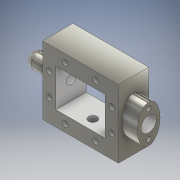
# Autodesk Inventor part: reverse gear steam chest
Saved by Autodesk Inventor 2017 (Build 210142000, 142)
## iProperties
Created: 2018-11-06
Part Number: reverse gear steam chest
Material: Generic
Document SubType Name: Modeling
Designer: User
Density: 1 g/cm^3
Appearance: Default
Author: User
Autodesk Inventor part; units mm, degrees
ref_plane "YZ Plane" through (0, 0, 0) normal (1, 0, 0) x (0, 1, 0)
ref_plane "XZ Plane" through (0, 0, 0) normal (0, 1, 0) x (-1, 0, 0)
ref_plane "XY Plane" through (0, 0, 0) normal (0, 0, 1) x (1, 0, 0)
sketch "Sketch1" plane through (0, 0, 0) normal (0, 1, 0) x (-1, 0, 0)
  line L0 (0, 0) -> (-40, 0)
  line L1 (-40, 0) -> (-40, -36)
  line L2 (-40, -36) -> (0, -36)
  line L3 (0, -36) -> (0, 0)
  line L4 (-7, -28) -> (-33, -28)
  line L5 (-33, -28) -> (-33, -8)
  line L6 (-33, -8) -> (-7, -8)
  line L7 (-7, -8) -> (-7, -28)
  dimension "d0" = 40
  dimension "d1" = 36
  dimension "d2" = 26
  constraints: 16 end point, 3 perpendicular, 2 parallel, 1 horizontal
  measures "d0" distance of L2.end L1.end
  measures "d1" distance of L1.end L0.end
  measures "d2" distance of L4.start L4.end
extrude "Extrusion1" add sketch "Sketch1" along normal blind 16
sketch "Sketch2" plane through (40, 0, 0) normal (1, 0, 0) x (0, 0, -1)
  line L0 (0, 0) -> (0, 16)
  line L1 (0, 8) -> (8, 8)
  line L2 (28, 0) -> (28, 16)
  line L3 (18, 14) -> (18, 2)
  ellipse E0 centre (18, 8) end of major axis (28, 8) minor radius 6
  line L4 (6.75, 0) -> (6.75, 16)
  line L5 (6.75, 8) -> (9.75, 8)
  circle A0 centre (11, 8) radius 1.25
  circle A1 centre (25, 8) radius 1.25
  circle A2 centre (18, 8) radius 2.5
  line L6 (12.25, 8) -> (15.5, 8)
  line L7 (20.5, 8) -> (23.75, 8)
  line L8 (20.5, 8) -> (23.75, 8)
  line L9 (26.25, 8) -> (28, 8)
  line L10 (8, 8) -> (9.75, 8)
  line L11 (12.25, 8) -> (15.5, 8)
  circle A3 centre (18, 8) radius 4
  line L12 (18, 8) -> (18, 10.5)
  line L13 (18, 12) -> (18, 14)
  dimension "d18" = 8
  dimension "d47" = 10
  dimension "d48" = 6
  dimension "d5" = 8
  dimension "d6" = 20
  dimension "d7" = 6
  dimension "d8" = 12
  dimension "d9" = 3
  dimension "d10" = 14
  dimension "d11" = 2.5
  dimension "d12" = 2.5
  dimension "d13" = 5
  dimension "d49" = 21.25
  dimension "d50" = 28
  dimension "d51" = 0
  dimension "d52" = 0
  dimension "d53" = 0
  dimension "d54" = 28
  dimension "d55" = 8
  dimension "d56" = 8
  dimension "d57" = 1.75
  dimension "d58" = 15.75
  dimension "d59" = 8
  dimension "d60" = 8
  dimension "d61" = 28
  dimension "d62" = 8
  constraints: 28 end point, 7 horizontal, 7 point on circle, 4 midpoint, 3 centre point, 3 parallel, 3 vertical, 2 coincident, 1 vertical alignment, 7 other
  measures "d5" distance of L1.start L1.end
  measures "d6" distance of L1.end L9.end
  measures "d7" distance of L12.start L3.start
  measures "d8" distance of L3.start L3.end
  measures "d9" distance of L5.start L5.end
  measures "d10" distance of L5.end L7.end
  measures "d11" diameter of A0
  measures "d12" diameter of A1
  measures "d13" diameter of A2
  measures "d49" distance between parallel lines of L4 L2
  measures "d50" distance between parallel lines of L0 L2
  measures "d51" distance between parallel lines of L9 L8
  measures "d52" distance between parallel lines of L9 L11
  measures "d53" distance between parallel lines of L1 L9
  measures "d54" distance from line of point (0, 0) L2
  measures "d55" distance from line of point (0, 0) L9
  measures "d56" distance from line of L2.end L9
  measures "d57" distance from line of L9.start L2
  measures "d58" distance from line of L6.start L2
  measures "d59" distance from line of L4.end L9
  measures "d60" distance from line of L0.end L9
  measures "d61" distance from line of point (0, 0) L2
  measures "d62" distance from line of point (0, 0) L9
extrude "Extrusion3" cut sketch "Sketch2" against normal blind 6 contours A1 | A0
extrude "Extrusion4" cut sketch "Sketch2" against normal blind 40 contours A2 L3 | L3 A2
extrude "Extrusion5" cut sketch "Sketch2" against normal blind 8 contours A3 L7 A2 L3 | L3 A2 L6 A3 | A3 L3 A2 L7 | L6 A2 L3 A3
extrude "Extrusion6" add sketch "Sketch2" along normal blind 8 contours E0 L9 A1 L7 A3 L3 | L3 A3 L6 A0 L5 E0 | E0 L3 A3 L7 A1 L9 | L5 A0 L6 A3 L3 E0
sketch "Sketch3" plane through (0, 0, 0) normal (0, -1, 0) x (1, 0, 0)
  line L0 (0, -20.5) -> (0, -15.5)
  line L1 (0, -18) -> (7, -18)
  line L2 (7, -8) -> (7, -28)
  line L3 (3.5, -18) -> (3.5, -12)
  line L4 (3.5, -12) -> (3.5, -24)
  line L5 (7, -28) -> (7, -36)
  line L6 (40, -36) -> (0, -36)
  line L7 (7, -32) -> (12, -32)
  line L8 (7, -8) -> (7, 0)
  line L9 (7, 0) -> (7, -4)
  line L10 (12, -4) -> (7, -4)
  circle A0 centre (12, -4) radius 1.5
  circle A1 centre (12, -32) radius 1.5
  circle A2 centre (3.5, -24) radius 1.5
  circle A3 centre (3.5, -12) radius 1.5
  line L11 (20, -36) -> (20, 0) construction
  line L12 (0, 0) -> (40, 0) construction
  circle A4 centre (28, -32) radius 1.5
  circle A5 centre (36.5, -24) radius 1.5
  circle A6 centre (36.5, -12) radius 1.5
  circle A7 centre (28, -4) radius 1.5
  dimension "d25" = 6
  dimension "d26" = 12
  dimension "d27" = 5
  dimension "d28" = 3
  dimension "d29" = 3
  dimension "d30" = 3
  dimension "d31" = 3
  dimension "d32" = 90
  dimension "d33" = 32
  dimension "d34" = 4
  dimension "d35" = 18
  dimension "d36" = 36
  dimension "d37" = 13
  dimension "d38" = 16.5
  dimension "d39" = 36
  dimension "d40" = 20
  dimension "d41" = 20
  dimension "d42" = 20
  dimension "d43" = 8
  dimension "d44" = 20.5
  constraints: 26 end point, 8 centre point, 7 midpoint, 5 parallel, 4 coincident, 4 symmetric about line, 3 vertical, 2 point on line, 1 horizontal, 1 perpendicular, 4 other
  measures "d25" distance of L3.start L3.end
  measures "d26" distance of L3.end L4.end
  measures "d27" distance of L7.start L7.end
  measures "d28" diameter of A0
  measures "d29" diameter of A1
  measures "d30" diameter of A2
  measures "d31" diameter of A3
  measures "d32" angle of L6 L2
  measures "d33" distance between parallel lines of L10 L6
  measures "d34" distance between parallel lines of L6 L7
  measures "d35" distance between parallel lines of L6 L1
  measures "d36" distance between parallel lines of L12 L6
  measures "d37" distance between parallel lines of L8 L11
  measures "d38" distance between parallel lines of L11 L3
  measures "d39" distance from line of point (0, 0) L6
  measures "d40" distance from line of point (0, 0) L11
  measures "d41" distance from line of L12.end L11
  measures "d42" distance from line of L6.start L11
  measures "d43" distance from line of A7.centre L11
  measures "d44" distance from line of L0.end L6
extrude "Extrusion7" cut sketch "Sketch3" against normal blind 16
sketch "Sketch4" plane through (0, 0, -36) normal (-1, 0, 0) x (0, 0, 1)
  circle A0 centre (18, 8) radius 4
  point P0 (36, 0)
  dimension "d63" = 8
  constraints: 1 centre point, 1 coincident
  measures "d63" diameter of A0
extrude "Extrusion9" add sketch "Sketch4" along normal blind 14
fillet "Fillet1" radius 4 1 edges at (-14, 8, -22)
sketch "Sketch6" plane through (40, 0, -36) normal (0, 0, -1) x (-1, 0, 0)
  line L0 (33, 5.5) -> (40, 5.5) projected
  circle A0 centre (19, 5.5) radius 2.25
  point P0 (40, 0)
  dimension "d73" = 4.5
  dimension "d74" = 21
  constraints: 1 centre point, 1 point on line
  measures "d73" diameter of A0
  measures "d74" distance of L0.end A0.centre
extrude "Extrusion11" cut sketch "Sketch6" against normal blind 10
body "Solid1"
